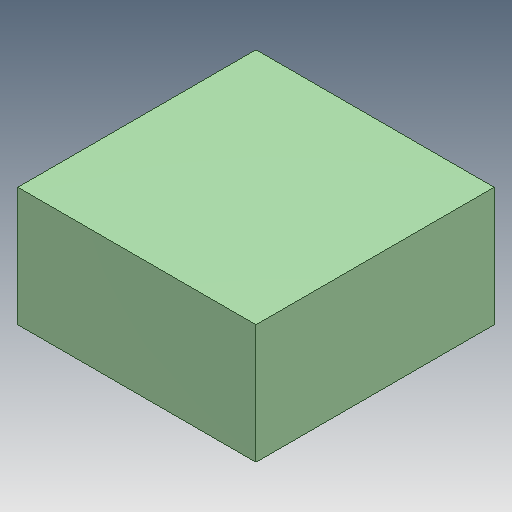
# Autodesk Inventor part: FIDUCIAL1X2_5
Saved by Autodesk Inventor 2017 (Build 210142000, 142)
## iProperties
Part Number: FIDUCIAL1X2_5
Material: Generisch
Document SubType Name: Modeling
Designer: Werkstatt
Density: 1 g/cm^3
Appearance: FIDUCIAL-1X2_5, FIDUCIAL1X2_5
Author: Werkstatt
Autodesk Inventor part; units mm, degrees
ref_plane "YZ Plane" through (0, 0, 0) normal (1, 0, 0) x (0, 1, 0)
ref_plane "XZ Plane" through (0, 0, 0) normal (0, 1, 0) x (-1, 0, 0)
ref_plane "XY Plane" through (0, 0, 0) normal (0, 0, 1) x (1, 0, 0)
sketch "FIDUCIAL-1X2_5, FIDUCIAL1X2_5_25" plane through (0, 0, 0) normal (0, 0, 1) x (1, 0, 0)
  line L0 (1, -1) -> (-1, -1)
  line L1 (-1, -1) -> (-1, 1)
  line L2 (-1, 1) -> (1, 1)
  line L3 (1, 1) -> (1, -1)
  constraints: 8 end point
extrude "Extrusion1" add sketch "FIDUCIAL-1X2_5, FIDUCIAL1X2_5_25" along normal blind 1
